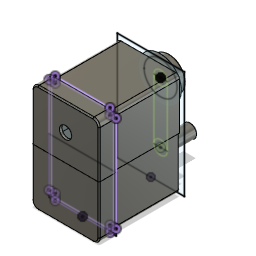
sharpener-exercise (Autodesk Fusion 360 design; units mm, degrees)
Autodesk Fusion 360 part; units mm, degrees
note: some values were not read from the file. Set by a fixed rule: which face or edge a step refers to.
sketch "Esquisse1" plane through (0, 0, 0) normal (0, 0, 1) x (1, 0, 0)
  line L0 (-27.5, 88.5) -> (27.5, 88.5)
  line L1 (27.5, 88.5) -> (27.5, 0)
  line L2 (27.5, 0) -> (-27.5, 0)
  line L3 (-27.5, 0) -> (-27.5, 88.5)
  dimension "d1" = 55
  dimension "d2" = 88.5
  constraint horizontal L0
  constraint vertical L1
  constraint horizontal L2
  constraint vertical L3
  constraint midpoint L2 origin
  measures "d1" distance of L0.start L0.end
  measures "d2" distance of L0.start L2.end
extrude "Extrusion1" add sketch "Esquisse1" along normal blind 56 makes body 1
fillet "Congé1" radius 5 4 edges at (-27.5, 88.5, 28) (27.5, 0, 28) (27.5, 88.5, 28) (-27.5, 0, 28) on bodies 1
shell "Coque1" thickness 2 removed faces 1 at (-9.1667, 31.1667, 56) on bodies 1
sketch "Esquisse2" plane through (0, 0, 56) normal (0, 0, 1) x (1, 0, 0)
  line L0 (-27.5, 45) -> (27.5, 45)
  line L1 (27.5, 45) -> (27.5, 0)
  line L2 (27.5, 0) -> (-27.5, 0)
  line L3 (-27.5, 0) -> (-27.5, 45)
  arc A0 (-22.5, 86.5) -> (-25.5, 83.5) centre (-22.5, 83.5) ccw
  line L4 (-22.5, 86.5) -> (22.5, 86.5)
  arc A1 (25.5, 83.5) -> (22.5, 86.5) centre (22.5, 83.5) ccw
  line L5 (25.5, 83.5) -> (25.5, 5)
  arc A2 (22.5, 2) -> (25.5, 5) centre (22.5, 5) ccw
  line L6 (22.5, 2) -> (-22.5, 2)
  arc A3 (-25.5, 5) -> (-22.5, 2) centre (-22.5, 5) ccw
  line L7 (-25.5, 5) -> (-25.5, 83.5)
  arc A4 (-27.5, 5) -> (-22.5, 0) centre (-22.5, 5) ccw
  line L8 (-22.5, 0) -> (22.5, 0)
  arc A5 (22.5, 0) -> (27.5, 5) centre (22.5, 5) ccw
  line L9 (27.5, 5) -> (27.5, 83.5)
  arc A6 (27.5, 83.5) -> (22.5, 88.5) centre (22.5, 83.5) ccw
  line L10 (22.5, 88.5) -> (-22.5, 88.5)
  arc A7 (-22.5, 88.5) -> (-27.5, 83.5) centre (-22.5, 83.5) ccw
  line L11 (-27.5, 83.5) -> (-27.5, 5)
  dimension "d8" = 55
  dimension "d9" = 45
  constraint horizontal L0
  constraint vertical L1
  constraint horizontal L2
  constraint vertical L3
  constraint midpoint L2 origin
  measures "d8" distance of L0.start L0.end
  measures "d9" distance of L0.start L2.end
extrude "Extrusion2" add sketch "Esquisse2" along normal blind 14 separate body contours L0 L1 L2 L3 L5 A2 L6 A3 L7 A4 L8 A5 L9 L11 | L0 L5 A2 L6 A3 L7 makes body 2
extrude "Extrusion3" add sketch "Esquisse2" against normal up to surface (54 mm away) contours L0 L5 A2 L6 A3 L7 bodies 2
shell "Coque2" thickness 2 removed faces 1 at (-8.5, 45, 20) on bodies 2
fillet "Congé3" radius 1 1 faces at (-9.1667, 31.1667, 0) on bodies 1
fillet "Congé4" radius 1 15 edges at (25.5, 25, 2) (24.6213, 2.8787, 2) (0, 2, 2) (-24.6213, 2.8787, 2) (-25.5, 25, 2) (-27.5, 25, 70) (-26.0355, 1.4645, 70) (0, 0, 70) (26.0355, 1.4645, 70) (27.5, 25, 70) (-25.5, 25, 58) (-24.6213, 2.8787, 58) (0, 2, 58) (24.6213, 2.8787, 58) (25.5, 25, 58) on bodies 2
fillet "Congé5" radius 0.5 5 edges at (-25.5, 25, 56) (-24.6213, 2.8787, 56) (0, 2, 56) (24.6213, 2.8787, 56) (25.5, 25, 56) on bodies 2
fillet "Congé6" radius 1 5 edges at (-23.5, 25, 58) (-23.2071, 4.2929, 58) (0, 4, 58) (23.2071, 4.2929, 58) (23.5, 25, 58) on bodies 2
fillet "Congé7" radius 1 5 edges at (-27.5, 25, 56) (-26.0355, 1.4645, 56) (0, 0, 56) (26.0355, 1.4645, 56) (27.5, 25, 56) on bodies 2
extrude "Extrusion4" add sketch "Esquisse2" along normal blind 14 separate body contours L0 A0 L4 A1 L5 L7 L9 A6 L10 A7 L11 | L0 A0 L4 A1 L5 L7 makes body 3
extrude "Extrusion5" add sketch "Esquisse2" against normal up to surface (54 mm away) contours L0 A0 L4 A1 L5 L7 bodies 3
shell "Coque3" thickness 2 removed faces 1 at (-8.5, 45, 20) on bodies 3
extrude "Extrusion6" cut 1 faces at (-7.5, 58.1667, 4) along direction (0, 0, -1) up to surface (2 mm away) on bodies 3 bodies 3
cylinder "CylindrePrimitive1" add diameter 12 height -40 placed x (1, 0, 0) y (0, 1, 0) z (0, 0, 1) at (0, 65, 70) bodies 3
delete_face "DeleteFace1" 1 faces at (-5.9925, 64.7009, 55.3333) on bodies 3
hole "Perçage2" at (0, 66.657, 70) direction (0, 0, -1) diameter 10 depth 18 tip angle 118 bodies 3
fillet "Congé8" radius 1 15 edges at (27.5, 64.25, 70) (26.0355, 87.0355, 70) (0, 88.5, 70) (-26.0355, 87.0355, 70) (-27.5, 64.25, 70) (27.5, 64.25, 56) (26.0355, 87.0355, 56) (0, 88.5, 56) (-26.0355, 87.0355, 56) (-27.5, 64.25, 56) (25.5, 64.25, 56) (24.6213, 85.6213, 56) (0, 86.5, 56) (-24.6213, 85.6213, 56) (-25.5, 64.25, 56) on bodies 3
fillet "Congé9" radius 2 5 edges at (23.5, 64.25, 58) (23.2071, 84.2071, 58) (0, 84.5, 58) (-23.2071, 84.2071, 58) (-23.5, 64.25, 58) on bodies 3
fillet "Congé10" radius 0.5 5 edges at (25.5, 64.25, 58) (24.6213, 85.6213, 58) (0, 86.5, 58) (-24.6213, 85.6213, 58) (-25.5, 64.25, 58) on bodies 3
sketch "Esquisse9" plane through (0, 0, 0) normal (0, 0, 1) x (1, 0, 0)
  circle A0 centre (0.0153, 66.5741) radius 17.5
  dimension "d48" = 35
  measures "d48" diameter of A0
extrude "Extrusion7" add sketch "Esquisse9" against normal blind 8 separate body makes body 4
sketch "Esquisse10" plane through (0, 0, -8) normal (0, 0, -1) x (-1, 0, 0)
  circle A0 centre (-0.0153, 66.5741) radius 17.5
  circle A1 centre (-0.0153, 66.5741) radius 13.5
  dimension "d51" = 27
  constraint concentric A0 A1
  measures "d51" diameter of A1
extrude "Extrusion8" add sketch "Esquisse10" along normal blind 7 contours A1 bodies 4
sketch "Esquisse11" plane through (0, 0, -8) normal (0, 0, -1) x (-1, 0, 0)
  circle A0 centre (-0.0153, 66.5741) radius 13.5
  circle A1 centre (-0.0153, 66.5741) radius 17.5
  line L0 (-5.5153, 66.5741) -> (5.4847, 66.5741)
  line L1 (5.4847, 66.5741) -> (5.4847, 17.0741)
  line L2 (5.4847, 17.0741) -> (-5.5153, 17.0741)
  line L3 (-5.5153, 17.0741) -> (-5.5153, 66.5741)
  circle A2 centre (-0.0153, 66.5741) radius 5.5
  circle A3 centre (-0.0153, 17.0741) radius 5.5
  line L4 (-0.0153, 66.5741) -> (-0.0153, 17.0741) construction
  point P0 (-0.0153, 66.5741)
  point P1 (-0.0153, 66.5741)
  point P2 (-0.0153, 66.5741)
  point P3 (-0.0153, 66.5741)
  point P4 (-290, 57)
  dimension "d54" = 11
  dimension "d55" = 49.5
  dimension "d56" = 11
  dimension "d57" = 11
  constraint horizontal L0
  constraint vertical L1
  constraint horizontal L2
  constraint vertical L3
  constraint midpoint L0 P3
  constraint midpoint L2 A3.centre
  constraint coincident P3 P2
  constraint coincident A3.centre L4.end
  measures "d54" distance of L0.start L0.end
  measures "d55" distance of L0.start L2.end
  measures "d56" diameter of A2
  measures "d57" diameter of A3
extrude "Extrusion9" add sketch "Esquisse11" along normal mid plane 4 from surface at 3.5 contours A0 L1 L3 A2 | A0 A1 L1 L3 | A1 L1 L3 A3 | L0 A2 | L0 A2 | L2 A3 | L2 A3 picked at (-0.7797, 55.7898) picked at (-0.0153, 50.4312) bodies 4
sketch "Esquisse12" plane through (0, 0, 0) normal (0, 0, 1) x (1, 0, 0)
  circle A0 centre (-0.0124, 16.9936) radius 5.5
  point P0 (0, 17)
  dimension "d61" = 11
  measures "d61" diameter of A0
extrude "Extrusion10" add sketch "Esquisse12" against normal blind 19 from surface at -13.5 bodies 4
sketch "Esquisse13" plane through (0, 0, -32.5) normal (0, 0, -1) x (-1, 0, 0)
  circle A0 centre (0.0124, 16.9936) radius 5.5
fillet "Congé11" radius 0.5 1 faces at (-1.5477, 18.2996, -32.5) on bodies 4
fillet "Congé12" radius 0.5 3 edges at (-16.3004, 60.2458, 0) (12.6017, 71.4559, -8) (12.6017, 61.6922, -15) 1 faces at (16.0665, 65.034, -8) on bodies 4
hidden bodies 1
named bodies: "boite", "tiroir", "taille crayon", "poignée"
